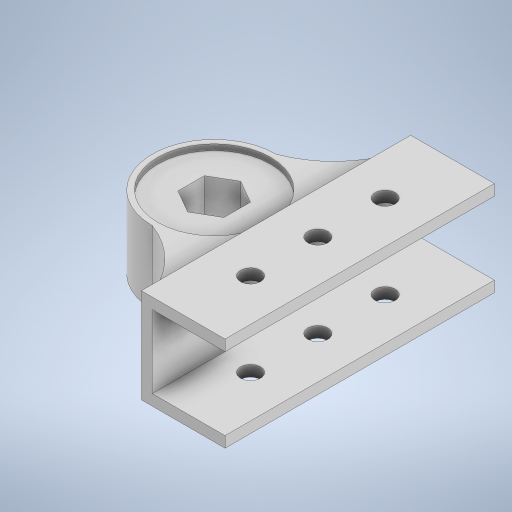
# Autodesk Inventor part: CH-1-01-BearingBracket
Saved by Autodesk Inventor 2023.1 (Build 271208000, 208)
## iProperties
Created: 2023-02-09
Part Number: CH-1-01-BearingBracket
Material: Generic
Document SubType Name: Modeling
Designer: eplym
Density: 1 g/cm^3
Appearance: Default
Author: eplym
Autodesk Inventor part; units mm, degrees
ref_plane "YZ Plane" through (0, 0, 0) normal (1, 0, 0) x (0, 1, 0)
ref_plane "XZ Plane" through (0, 0, 0) normal (0, 1, 0) x (-1, 0, 0)
ref_plane "XY Plane" through (0, 0, 0) normal (0, 0, 1) x (1, 0, 0)
sketch "Sketch1" plane through (0, 0, 0) normal (0, 1, 0) x (-1, 0, 0)
  circle A0 centre (0, 0) radius 17
  dimension "d6" = 34
  constraints: 1 centre point, 1 coincident
  measures "d6" diameter of A0
extrude "Extrusion1" add sketch "Sketch1" along normal blind 19.98
sketch "Sketch2" plane through (0, 19.98, 0) normal (0, 1, 0) x (1, 0, 0)
  circle A0 centre (0, 0) radius 15.5
  dimension "d9" = 31
  constraints: 1 centre point, 1 coincident
  measures "d9" diameter of A0
extrude "Extrusion2" cut sketch "Sketch2" against normal blind 1.61
sketch "Sketch4" plane through (0, 0, 0) normal (0, -1, 0) x (1, 0, 0)
  circle A0 centre (0, 0) radius 15.5
  dimension "d15" = 31
  constraints: 1 centre point, 1 coincident
  measures "d15" diameter of A0
extrude "Extrusion4" cut sketch "Sketch4" against normal blind 1.61
sketch "Sketch5" plane through (0, 0, 0) normal (0, -1, 0) x (1, 0, 0)
  circle A0 centre (0, 0) radius 17 projected
  line L0 (17, 0) -> (17, 17)
  line L1 (17, 17) -> (17, 37)
  line L2 (17, 0) -> (17, -17)
  line L3 (17, -17) -> (17, -37)
  line L4 (17, 37) -> (37, 37)
  line L5 (37, 37) -> (37, -37)
  line L6 (37, -37) -> (17, -37)
  arc A1 (0, 17) -> (17, 37) centre (-9.2645, 42.0999) ccw
  circle A2 centre (0, 0) radius 14.285 projected
  arc A3 (17, -37) -> (0, -17) centre (-9.2645, -42.0999) ccw
  point P0 (0, -17)
  dimension "d18" = 20
  dimension "d19" = 20
  dimension "d20" = 20
  constraints: 14 end point, 6 point on circle, 3 point on line, 2 centre point, 2 perpendicular, 2 tangent, 1 horizontal, 1 vertical
  measures "d18" distance of L0.end L1.end
  measures "d19" distance of L2.end L3.end
  measures "d20" distance of L1.end L4.end
extrude "Extrusion5" add sketch "Sketch5" against normal blind 19.98 contours L2 L3 A3 A0 | A0 A1 L1 L0 | L0 L1 L4 L5 L6 L3 L2
sketch "Sketch7" plane through (0, 19.98, 0) normal (0, 1, 0) x (1, 0, 0)
  arc A0 (0, 17) -> (17, 37) centre (-9.2645, 42.0999) ccw projected
  line L0 (37, -37) -> (37, 37) projected
  line L1 (17, 37) -> (37, 37)
  line L2 (37, 37) -> (37, -37)
  line L3 (37, -37) -> (17, -37)
  line L4 (17, -37) -> (17, 37)
  point P0 (0, 0)
  constraints: 8 end point, 2 parallel, 1 horizontal, 1 perpendicular
extrude "Extrusion6" add sketch "Sketch7" along normal blind 3
sketch "Sketch9" plane through (0, 0, 0) normal (0, -1, 0) x (1, 0, 0)
  line L0 (17, 37) -> (37, 37) projected
  line L1 (17, -37) -> (17, 37) projected
  line L2 (37, 37) -> (17, 37)
  line L3 (17, 37) -> (17, -37)
  line L4 (17, -37) -> (37, -37)
  line L5 (37, -37) -> (37, 37)
  point P0 (0, 0)
  constraints: 8 end point, 2 parallel, 1 horizontal, 1 perpendicular
extrude "Extrusion7" add sketch "Sketch9" along normal blind 3
sketch "Sketch11" plane through (37, 22.98, 37) normal (1, 0, 0) x (0, 0, -1)
  line L0 (0, -3) -> (0, 0) projected
  line L1 (74, -22.98) -> (74, -25.98) projected
  line L2 (0, 0) -> (74, 0)
  line L3 (74, 0) -> (74, -25.98)
  line L4 (74, -25.98) -> (0, -25.98)
  line L5 (0, -25.98) -> (0, 0)
  point P0 (37, -22.98)
  constraints: 8 end point, 2 parallel, 1 horizontal, 1 perpendicular
extrude "Extrusion8" add sketch "Sketch11" along normal blind 3
sketch "Sketch12" plane through (17, 19.98, 37) normal (0, 0, 1) x (1, 0, 0)
  line L0 (23, -22.98) -> (23, 3) projected
  line L1 (23, 0) -> (3, 0)
  line L2 (3, 0) -> (3, -19.98)
  line L3 (3, -19.98) -> (23, -19.98)
  line L4 (23, -19.98) -> (23, 0)
  line L5 (0, 3) -> (23, 3) projected
  line L6 (0, -19.98) -> (0, 0) projected
  line L7 (0, -22.98) -> (23, -22.98) projected
  point P0 (-17, -19.98)
  point P1 (23, -19.98)
  dimension "d29" = 3
  dimension "d30" = 3
  dimension "d31" = 3
  constraints: 8 end point, 2 parallel, 1 horizontal, 1 perpendicular, 1 point on line
  measures "d29" distance between parallel lines of L5 L1
  measures "d30" distance between parallel lines of L6 L2
  measures "d31" distance between parallel lines of L7 L3
extrude "Extrusion9" cut sketch "Sketch12" against normal through all
sketch "Sketch13" plane through (0, 18.37, 0) normal (0, 1, 0) x (1, 0, 0)
  line L0 (0, 7.29) -> (6.3133, 3.645)
  line L1 (6.3133, 3.645) -> (6.3133, -3.645)
  line L2 (6.3133, -3.645) -> (0, -7.29)
  line L3 (0, -7.29) -> (-6.3133, -3.645)
  line L4 (-6.3133, -3.645) -> (-6.3133, 3.645)
  line L5 (-6.3133, 3.645) -> (0, 7.29)
  point P0 (0, 0)
  point P1 (0, 0)
  constraints: 12 end point, 13 other
extrude "Extrusion10" cut sketch "Sketch13" against normal through all
sketch "Sketch14" plane through (0, 22.98, 0) normal (0, 1, 0) x (1, 0, 0)
  line L0 (40, 37) -> (40, -37) projected
  line L1 (17, -37) -> (40, -37) projected
  point P0 (0, 0)
  point P1 (28.5, 0)
  dimension "d37" = 11.5
  dimension "d38" = 37
  measures "d37" distance from line of L0 point (28.5, 0)
  measures "d38" distance from line of L1 point (28.5, 0)
hole "Hole1" at (28.5, 22.98, 0) direction (0, -1, 0) diameter 5.5 end through all clearance for "Flat Head Machine Screw" size "M5" standard "Ansi Metric M Profile"
sketch "Sketch15" plane through (0, 22.98, 0) normal (0, 1, 0) x (1, 0, 0)
  circle A0 centre (28.5, -18.5) radius 3.0917
  circle A1 centre (28.5, 18.5) radius 2.226
  line L0 (17, 37) -> (40, 37) projected
  line L1 (17, -37) -> (40, -37) projected
  point P0 (0, 0)
  point P1 (28.5, 37)
  dimension "d47" = 18.5
  dimension "d48" = 18.5
  constraints: 2 centre point, 1 midpoint
  measures "d47" distance from line of L0 A1.centre
  measures "d48" distance from line of L1 A0.centre
hole "Hole2" at (28.5, 22.98, 18.5) at (28.5, 22.98, -18.5) direction (0, -1, 0) diameter 5.5 end through all clearance for "Flat Head Machine Screw" size "M5" standard "Ansi Metric M Profile"
body "Solid1"
